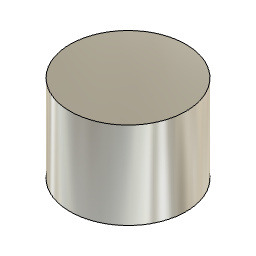
crane assembly v9 (Autodesk Fusion 360 archive; units mm, degrees)
design "electromagnet"
Autodesk Fusion 360 part; units mm, degrees
sketch "Sketch1" plane through (0, 0, 0) normal (0, 0, 1) x (1, 0, 0)
  circle A0 centre (0, 0) radius 10
  dimension "d1" = 20
  constraint coincident A0.centre origin
  measures "d1" diameter of A0
extrude "Extrude1" add sketch "Sketch1" along normal blind 15
sketch "Sketch2" plane through (0, 0, 0) normal (0, 0, -1) x (1, 0, 0)
  circle A0 centre (0, 0) radius 10
  circle A1 centre (0, 0) radius 2
  dimension "d4" = 4
  constraint concentric A0 A1
  measures "d4" diameter of A1
extrude "Extrude2" cut sketch "Sketch2" against normal blind 5 contours A1

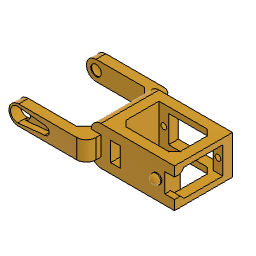
design "second link"
Autodesk Fusion 360 part; units mm, degrees
sketch "Sketch1" plane through (0, 0, 0) normal (0, 0, 1) x (1, 0, 0)
  line L0 (0, 0) -> (40, 0)
  line L1 (40, 0) -> (40, 5)
  line L2 (40, 5) -> (0, 5)
  line L3 (0, 5) -> (0, 0)
  dimension "d1" = 40
  dimension "d2" = 5
  constraint horizontal L0
  constraint vertical L1
  constraint horizontal L2
  constraint vertical L3
  constraint coincident L0.start L3.end
  measures "d1" distance of L0.start L0.end
  measures "d2" distance of L0.start L2.end
extrude "Extrude1" add sketch "Sketch1" along normal blind 10
sketch "Sketch3" plane through (0, 0, 0) normal (0, -1, 0) x (1, 0, 0)
  line L0 (0, 0) -> (40, 0)
  line L1 (40, 0) -> (40, 10)
  line L2 (40, 10) -> (0, 10)
  line L3 (0, 10) -> (0, 0)
  line L4 (0, 5) -> (4.5, 5) construction
  circle A0 centre (4.5, 5) radius 3.7
  line L5 (4.5, 5) -> (18.5, 5) construction
  circle A1 centre (18.5, 5) radius 2.25
  line L6 (18.5, 5) -> (18.5, 7.25) construction
  line L7 (18.5, 5) -> (18.5, 2.75) construction
  line L8 (4.5, 5) -> (4.5, 8.7) construction
  line L9 (4.5, 5) -> (4.5, 1.3) construction
  line L10 (4.5, 1.3) -> (18.5, 2.75)
  line L11 (4.5, 8.7) -> (18.5, 7.25)
  dimension "d5" = 4.5
  dimension "d6" = 7.4
  dimension "d7" = 14
  dimension "d8" = 4.5
  constraint midpoint L3 L4.start
  constraint perpendicular L3 L4
  constraint coincident L4.end A0.centre
  constraint parallel L4 L5
  constraint coincident L5.end A1.centre
  constraint coincident A1 L6.end
  constraint perpendicular L5 L6
  constraint coincident A1 L7.end
  constraint perpendicular L5 L7
  constraint coincident A0 L8.end
  constraint perpendicular L5 L8
  constraint coincident A0 L9.end
  constraint perpendicular L5 L9
  measures "d5" distance of L4.start L4.end
  measures "d6" diameter of A0
  measures "d7" distance of L4.end L5.end
  measures "d8" diameter of A1
extrude "Extrude2" cut sketch "Sketch3" against normal blind 5 contours A0 L10 L11
extrude "Extrude3" cut sketch "Sketch3" against normal blind 3 contours A0 A1 L10 L11 | A1
fillet "Fillet1" radius 5 2 edges at (0, 2.5, 10) (0, 2.5, 0)
sketch "Sketch4" plane through (0, 5, 0) normal (0, 1, 0) x (-1, 0, 0)
  arc A0 (-5.2583, 8.6215) -> (-5.2583, 1.3785) centre (-4.5, 5) ccw
  line L0 (-5.2583, 8.6215) -> (-4.5, 8.7)
  arc A1 (-4.5, 1.3) -> (-4.5, 8.7) centre (-4.5, 5) ccw
  line L1 (-4.5, 1.3) -> (-5.2583, 1.3785)
  arc A2 (-5, 0) -> (-5, 10) centre (-5, 5) ccw
  line L2 (-5, 10) -> (-40, 10)
  line L3 (-40, 10) -> (-40, 0)
  line L4 (-40, 0) -> (-5, 0)
  line L5 (-40, 0) -> (-35, 0)
  line L6 (-35, 0) -> (-35, 10)
  line L7 (-35, 10) -> (-40, 10)
  line L8 (-40, 10) -> (-40, 0)
  dimension "d15" = 5
  constraint horizontal L5
  constraint vertical L6
  constraint horizontal L7
  constraint vertical L8
  constraint coincident L3.end L4.start
  measures "d15" distance of L3.end L5.end
extrude "Extrude4" add sketch "Sketch4" along normal blind 40 contours L2 L3 L4 L5 L6 L7 L8
sketch "Sketch5" plane through (35, 0, 0) normal (-1, 0, 0) x (0, -1, 0)
  line L0 (-5, 0) -> (-5, 10)
  line L1 (-5, 10) -> (-45, 10)
  line L2 (-45, 10) -> (-45, 0)
  line L3 (-45, 0) -> (-5, 0)
  line L4 (-45, 10) -> (-40, 10)
  line L5 (-40, 10) -> (-40, 0)
  line L6 (-40, 0) -> (-45, 0)
  line L7 (-45, 0) -> (-45, 10)
  dimension "d18" = 5
  constraint horizontal L4
  constraint vertical L5
  constraint horizontal L6
  constraint vertical L7
  constraint coincident L1.end L2.start
  measures "d18" distance of L1.end L4.end
extrude "Extrude5" add sketch "Sketch5" along normal blind 35 contours L1 L2 L3 L4 L5 L6 L7
sketch "Sketch6" plane through (0, 40, 0) normal (0, -1, 0) x (1, 0, 0)
  line L0 (35, 0) -> (35, 10)
  line L1 (35, 10) -> (0, 10)
  line L2 (0, 10) -> (0, 0)
  line L3 (0, 0) -> (35, 0)
  line L4 (0, 5) -> (5, 5) construction
  circle A0 centre (5, 5) radius 2.75
  dimension "d21" = 5
  dimension "d22" = 5.5
  constraint midpoint L2 L4.start
  constraint perpendicular L2 L4
  constraint coincident L4.end A0.centre
  measures "d21" distance of L4.start L4.end
  measures "d22" diameter of A0
extrude "Extrude6" cut sketch "Sketch6" against normal blind 3 contours A0
fillet "Fillet2" radius 2.5 1 edges at (2.4361, 43, 5.9944)
fillet "Fillet3" radius 5 2 edges at (0, 42.5, 10) (0, 42.5, 0)
chamfer "Chamfer1" distance 5 angle 45 2 edges at (35, 40, 5) (35, 5, 5)
sketch "Sketch7" plane through (40, 0, 0) normal (1, 0, 0) x (0, 1, 0)
  line L0 (0, 0) -> (45, 0)
  line L1 (45, 0) -> (45, 10)
  line L2 (45, 10) -> (0, 10)
  line L3 (0, 10) -> (0, 0)
  line L4 (45, 10) -> (32.5, 10) construction
  line L5 (32.5, 10) -> (12.5, 10)
  line L6 (12.5, 10) -> (12.5, 0)
  line L7 (12.5, 0) -> (32.5, 0)
  line L8 (32.5, 0) -> (32.5, 10)
  line L9 (32.5, 10) -> (12.5, 10)
  line L10 (12.5, 10) -> (12.5, 15)
  line L11 (12.5, 15) -> (32.5, 15)
  line L12 (32.5, 15) -> (32.5, 10)
  line L13 (32.5, 0) -> (12.5, 0)
  line L14 (12.5, 0) -> (12.5, -5)
  line L15 (12.5, -5) -> (32.5, -5)
  line L16 (32.5, -5) -> (32.5, 0)
  line L17 (32.5, -5) -> (37.5, -5)
  line L18 (37.5, -5) -> (37.5, 15)
  line L19 (37.5, 15) -> (32.5, 15)
  line L20 (32.5, 15) -> (32.5, -5)
  line L21 (12.5, -5) -> (7.5, -5)
  line L22 (7.5, -5) -> (7.5, 15)
  line L23 (7.5, 15) -> (12.5, 15)
  line L24 (12.5, 15) -> (12.5, -5)
  dimension "d30" = 12.5
  dimension "d31" = 20
  dimension "d32" = 5
  dimension "d33" = 20
  dimension "d34" = 5
  dimension "d35" = 5
  dimension "d36" = 20
  dimension "d37" = 5
  dimension "d38" = 20
  constraint coincident L1.end L2.start
  constraint perpendicular L1 L4
  constraint horizontal L5
  constraint vertical L6
  constraint horizontal L7
  constraint vertical L8
  constraint coincident L0 L6.end
  constraint horizontal L9
  constraint vertical L10
  constraint horizontal L11
  constraint vertical L12
  constraint horizontal L13
  constraint vertical L14
  constraint horizontal L15
  constraint vertical L16
  constraint horizontal L17
  constraint vertical L18
  constraint horizontal L19
  constraint vertical L20
  constraint horizontal L21
  constraint vertical L22
  constraint horizontal L23
  constraint vertical L24
  measures "d30" distance of L1.end L4.end
  measures "d31" distance of L4.end L5.end
  measures "d32" distance of L4.end L11.end
  measures "d33" distance of L7.end L6.end
  measures "d34" distance of L7.end L15.end
  measures "d35" distance of L15.end L17.end
  measures "d36" distance of L15.end L11.end
  measures "d37" distance of L14.end L21.end
  measures "d38" distance of L14.end L10.end
extrude "Extrude7" add sketch "Sketch7" along normal blind 5 contours L0 L2 L5 L6 L7 L8 L9 L13 L20 L24 | L0 L14 L21 L22 L24 | L0 L2 L6 L22 L24 | L0 L7 L13 L14 L15 L16 L20 L24 | L0 L2 L8 L18 L20 | L0 L16 L17 L18 L20 | L2 L5 L9 L10 L11 L12 L20 L24 | L2 L10 L22 L23 L24 | L2 L12 L18 L19 L20
revolve "Revolve1" add 2 faces at (40, 17.5, 13.3333) (40, 17.5, 13.3333) angle 360 about axis through (40, 0, 10) along (0, 1, 0)
revolve "Revolve2" add 2 faces at (40, 17.5, -1.6667) (40, 17.5, -1.6667) angle 360 about axis through (40, 0, 0) along (0, 1, 0)
sketch "Sketch8" plane through (45, 0, 0) normal (1, 0, 0) x (0, 1, 0)
  line L0 (37.5, -5) -> (37.5, 15)
  line L1 (37.5, 15) -> (7.5, 15)
  line L2 (7.5, 15) -> (7.5, -5)
  line L3 (7.5, -5) -> (37.5, -5)
  line L4 (37.5, 15) -> (32.5, 15)
  line L5 (32.5, 15) -> (32.5, 12)
  line L6 (32.5, 12) -> (37.5, 12)
  line L7 (37.5, 12) -> (37.5, 15)
  line L8 (37.5, -5) -> (32.5, -5)
  line L9 (32.5, -5) -> (32.5, -2)
  line L10 (32.5, -2) -> (37.5, -2)
  line L11 (37.5, -2) -> (37.5, -5)
  line L12 (7.5, -5) -> (12.5, -5)
  line L13 (12.5, -5) -> (12.5, 0)
  line L14 (12.5, 0) -> (7.5, 0)
  line L15 (7.5, 0) -> (7.5, -5)
  line L16 (7.5, 15) -> (12.5, 15)
  line L17 (12.5, 15) -> (12.5, 10)
  line L18 (12.5, 10) -> (7.5, 10)
  line L19 (7.5, 10) -> (7.5, 15)
  dimension "d43" = 5
  dimension "d44" = 3
  dimension "d45" = 5
  dimension "d46" = 3
  dimension "d47" = 5
  dimension "d48" = 5
  dimension "d49" = 5
  dimension "d50" = 5
  constraint horizontal L4
  constraint vertical L5
  constraint horizontal L6
  constraint vertical L7
  constraint coincident L0.end L1.start
  constraint horizontal L8
  constraint vertical L9
  constraint horizontal L10
  constraint vertical L11
  constraint coincident L0.start L3.end
  constraint horizontal L12
  constraint vertical L13
  constraint horizontal L14
  constraint vertical L15
  constraint coincident L2.end L3.start
  constraint horizontal L16
  constraint vertical L17
  constraint horizontal L18
  constraint vertical L19
  constraint coincident L1.end L2.start
  measures "d43" distance of L0.end L4.end
  measures "d44" distance of L0.end L6.end
  measures "d45" distance of L0.start L8.end
  measures "d46" distance of L0.start L10.end
  measures "d47" distance of L2.end L12.end
  measures "d48" distance of L2.end L14.end
  measures "d49" distance of L1.end L16.end
  measures "d50" distance of L1.end L18.end
extrude "Extrude8" add sketch "Sketch8" along normal blind 33 contours L0 L3 L8 L9 L10 L11 | L0 L1 L4 L5 L6 L7 | L2 L3 L12 L13 L14 L15 | L1 L2 L16 L17 L18 L19
sketch "Sketch9" plane through (0, 0, -2) normal (0, 0, 1) x (-1, 0, 0)
  line L0 (-45, -37.5) -> (-45, -32.5)
  line L1 (-45, -32.5) -> (-78, -32.5)
  line L2 (-78, -32.5) -> (-78, -37.5)
  line L3 (-78, -37.5) -> (-45, -37.5)
  line L4 (-45, -32.5) -> (-50, -32.5)
  line L5 (-50, -32.5) -> (-50, -37.5)
  line L6 (-50, -37.5) -> (-45, -37.5)
  line L7 (-45, -37.5) -> (-45, -32.5)
  line L8 (-78, -37.5) -> (-73, -37.5)
  line L9 (-73, -37.5) -> (-73, -32.5)
  line L10 (-73, -32.5) -> (-78, -32.5)
  line L11 (-78, -32.5) -> (-78, -37.5)
  dimension "d53" = 5
  dimension "d54" = 5
  dimension "d55" = 5
  dimension "d56" = 5
  constraint horizontal L4
  constraint vertical L5
  constraint horizontal L6
  constraint vertical L7
  constraint coincident L0.end L1.start
  constraint horizontal L8
  constraint vertical L9
  constraint horizontal L10
  constraint vertical L11
  constraint coincident L2.end L3.start
  measures "d53" distance of L0.end L4.end
  measures "d54" distance of L0.end L0.start
  measures "d55" distance of L2.end L8.end
  measures "d56" distance of L2.end L1.end
extrude "Extrude9" add sketch "Sketch9" along normal blind 14 contours L0 L1 L3 L4 L5 L6 L7 | L1 L2 L3 L8 L9 L10 L11
sketch "Sketch10" plane through (0, 32.5, 0) normal (0, -1, 0) x (1, 0, 0)
  line L0 (73, 12) -> (73, -2)
  line L1 (73, -2) -> (50, -2)
  line L2 (50, -2) -> (50, 12)
  line L3 (45, 15) -> (45, -5)
  line L4 (45, -5) -> (78, -5)
  line L5 (78, -5) -> (78, 15)
  line L6 (45, 5) -> (47.5, 5)
  circle A0 centre (47.5, 5) radius 1.5
  line L7 (73, 5) -> (75.5, 5)
  circle A1 centre (75.5, 5) radius 1.5
  line L8 (50, 12) -> (73, 12)
  line L9 (78, 15) -> (45, 15)
  dimension "d59" = 2.5
  dimension "d60" = 3
  dimension "d61" = 2.5
  dimension "d62" = 3
  constraint midpoint L3 L6.start
  constraint perpendicular L2 L6
  constraint coincident L6.end A0.centre
  constraint midpoint L0 L7.start
  constraint perpendicular L5 L7
  constraint coincident L7.end A1.centre
  measures "d59" distance of L6.start L6.end
  measures "d60" diameter of A0
  measures "d61" distance of L7.start L7.end
  measures "d62" diameter of A1
extrude "Extrude10" cut sketch "Sketch10" against normal blind 5 contours A0 | A1
sketch "Sketch11" plane through (0, 32.5, 0) normal (0, -1, 0) x (1, 0, 0)
  circle A0 centre (47.5, 5) radius 1.5
  circle A1 centre (75.5, 5) radius 1.5
  line L0 (73, 12) -> (73, -2)
  line L1 (73, -2) -> (50, -2)
  line L2 (50, -2) -> (50, 12)
  line L3 (45, 15) -> (45, -5)
  line L4 (45, -5) -> (78, -5)
  line L5 (78, -5) -> (78, 15)
  line L6 (78, 15) -> (73, 15)
  line L7 (73, 15) -> (73, 12)
  line L8 (73, 12) -> (78, 12)
  line L9 (78, 12) -> (78, 15)
  line L10 (78, -5) -> (73, -5)
  line L11 (73, -5) -> (73, -2)
  line L12 (73, -2) -> (78, -2)
  line L13 (78, -2) -> (78, -5)
  line L14 (50, 12) -> (73, 12)
  line L15 (78, 15) -> (45, 15)
  dimension "d69" = 5
  dimension "d70" = 3
  dimension "d71" = 5
  dimension "d72" = 3
  constraint horizontal L6
  constraint vertical L7
  constraint horizontal L8
  constraint vertical L9
  constraint coincident L5.end L6.start
  constraint horizontal L10
  constraint vertical L11
  constraint horizontal L12
  constraint vertical L13
  constraint coincident L4.end L5.start
  measures "d69" distance of L5.end L6.end
  measures "d70" distance of L5.end L8.end
  measures "d71" distance of L4.end L10.end
  measures "d72" distance of L4.end L12.end
extrude "Extrude11" add sketch "Sketch11" along normal blind 20 contours L5 L6 L7 L8 L9 L15 | L4 L5 L10 L11 L12 L13
sketch "Sketch12" plane through (0, 0, 0) normal (0, 0, 1) x (-1, 0, 0)
  line L0 (-45, -12.5) -> (-45, -7.5)
  line L1 (-45, -7.5) -> (-78, -7.5)
  line L2 (-78, -7.5) -> (-78, -12.5)
  line L3 (-78, -12.5) -> (-45, -12.5)
  line L4 (-78, -7.5) -> (-73, -7.5) construction
  line L5 (-73, -7.5) -> (-73, -12.5) construction
  line L6 (-73, -12.5) -> (-78, -12.5) construction
  line L7 (-78, -12.5) -> (-78, -7.5) construction
  line L8 (-45, -7.5) -> (-50, -7.5) construction
  line L9 (-50, -7.5) -> (-50, -12.5) construction
  line L10 (-50, -12.5) -> (-45, -12.5) construction
  line L11 (-45, -12.5) -> (-45, -7.5) construction
  line L12 (-73, -7.5) -> (-50, -7.5)
  line L13 (-50, -7.5) -> (-50, -12.5)
  line L14 (-50, -12.5) -> (-73, -12.5)
  line L15 (-73, -12.5) -> (-73, -7.5)
  dimension "d75" = 5
  dimension "d76" = 5
  constraint horizontal L4
  constraint vertical L5
  constraint horizontal L6
  constraint vertical L7
  constraint coincident L1.end L2.start
  constraint horizontal L8
  constraint vertical L9
  constraint horizontal L10
  constraint vertical L11
  constraint coincident L0.end L1.start
  constraint horizontal L12
  constraint vertical L13
  constraint horizontal L14
  constraint vertical L15
  measures "d75" distance of L1.end L4.end
  measures "d76" distance of L0.end L8.end
extrude "Extrude12" add sketch "Sketch12" along normal blind 10 contours L1 L3 L12 L13 L14 L15
chamfer "Chamfer2" distance 2 angle 45 2 edges at (75.5, 12.5, 0) (75.5, 12.5, 10)
chamfer "Chamfer3" distance 3 angle 45 6 edges at (73, 12.5, 13.5) (73, 32.5, 13.5) (45, 12.5, 12.5) (45, 12.5, -2.5) (73, 32.5, -3.5) (73, 12.5, -3.5)
fillet "Fillet4" radius 5 2 edges at (40, 0, 5) (40, 45, 5)
sketch "Sketch13" plane through (0, 7.5, 0) normal (0, -1, 0) x (1, 0, 0)
  line L0 (73, 10) -> (78, 10)
  line L1 (78, 10) -> (78, 15)
  line L2 (78, 15) -> (40, 15)
  arc A0 (40, 15) -> (35, 10) centre (40, 10) ccw
  line L3 (35, 10) -> (40, 10)
  line L4 (40, 10) -> (40, 0)
  line L5 (40, 0) -> (35, 0)
  arc A1 (35, 0) -> (40, -5) centre (40, 0) ccw
  line L6 (40, -5) -> (78, -5)
  line L7 (78, -5) -> (78, 0)
  line L8 (78, 0) -> (73, 0)
  line L9 (73, 0) -> (73, 10)
  line L10 (50, 10) -> (50, 0)
  line L11 (50, 0) -> (45, 0)
  line L12 (45, 0) -> (45, 10)
  line L13 (45, 10) -> (50, 10)
  line L14 (73, 5) -> (69, 5) construction
  circle A2 centre (69, 5) radius 2.5
  dimension "d83" = 4
  dimension "d84" = 5
  constraint midpoint L9 L14.start
  constraint perpendicular L9 L14
  constraint coincident L14.end A2.centre
  measures "d83" distance of L14.start L14.end
  measures "d84" diameter of A2
extrude "Extrude13" add sketch "Sketch13" along normal blind 3 contours A2
fillet "Fillet5" radius 2.5 1 edges at (66.6692, 4.5, 4.096)

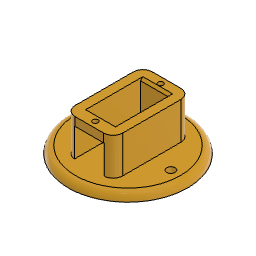
design "crane_base"
Autodesk Fusion 360 part; units mm, degrees
sketch "Sketch1" plane through (0, 0, 0) normal (0, 0, 1) x (1, 0, 0)
  circle A0 centre (0, 0) radius 25
  line L0 (0, 0) -> (-18, 0) construction
  line L1 (0, 0) -> (18, 0) construction
  circle A1 centre (-18, 0) radius 1.75
  circle A2 centre (18, 0) radius 1.75
  dimension "d1" = 50
  dimension "d25" = 18
  dimension "d26" = 18
  dimension "d27" = 3.5
  dimension "d28" = 3.5
  constraint coincident A0.centre L0.start
  constraint horizontal L0
  constraint parallel L0 L1
  constraint coincident L0.end A1.centre
  constraint coincident L1.end A2.centre
  measures "d1" diameter of A0
  measures "d25" distance of A0.centre L0.end
  measures "d26" distance of A0.centre L1.end
  measures "d27" diameter of A1
  measures "d28" diameter of A2
extrude "Extrude1" add sketch "Sketch1" along normal blind 3
sketch "Sketch2" plane through (0, 0, 3) normal (0, 0, 1) x (-1, 0, 0)
  circle A0 centre (0, 0) radius 25
  line L0 (-6.25, 11.5) -> (6.25, 11.5)
  line L1 (6.25, 11.5) -> (6.25, -11.5)
  line L2 (6.25, -11.5) -> (-6.25, -11.5)
  line L3 (-6.25, -11.5) -> (-6.25, 11.5)
  line L4 (-6.25, 11.5) -> (6.25, -11.5) construction
  line L5 (6.25, 11.5) -> (-6.25, -11.5) construction
  line L6 (-10, -16.225) -> (10, -16.225)
  line L7 (10, -16.225) -> (10, 16.225)
  line L8 (10, 16.225) -> (-10, 16.225)
  line L9 (-10, 16.225) -> (-10, -16.225)
  line L10 (-10, -16.225) -> (10, 16.225) construction
  line L11 (10, -16.225) -> (-10, 16.225) construction
  circle A1 centre (-18, 0) radius 1.75
  circle A2 centre (18, 0) radius 1.75
  dimension "d4" = 12.5
  dimension "d5" = 23
  dimension "d6" = 20
  dimension "d7" = 32.45
  constraint horizontal L0
  constraint perpendicular L0 L1
  constraint parallel L0 L2
  constraint parallel L1 L3
  constraint coincident L4 A0.centre
  constraint coincident L5 A0.centre
  constraint coincident A0.centre origin
  constraint horizontal L6
  constraint perpendicular L6 L7
  constraint parallel L6 L8
  constraint parallel L7 L9
  constraint coincident L10 A0.centre
  constraint coincident L11 A0.centre
  measures "d4" distance of L1.end L2.end
  measures "d5" distance of L0.end L1.end
  measures "d6" distance of L7.end L8.end
  measures "d7" distance of L6.end L7.end
extrude "Extrude2" add sketch "Sketch2" along normal blind 15.55 contours L6 L7 L8 L9
sketch "Sketch3" plane through (0, 0, 18.55) normal (0, 0, 1) x (-1, 0, 0)
  line L0 (6.25, -11.5) -> (-6.25, -11.5)
  line L1 (-6.25, -11.5) -> (-6.25, 11.5)
  line L2 (-6.25, 11.5) -> (6.25, 11.5)
  line L3 (6.25, 11.5) -> (6.25, -11.5)
  line L4 (-10, 16.225) -> (-10, -16.225)
  line L5 (-10, -16.225) -> (10, -16.225)
  line L6 (10, -16.225) -> (10, 16.225)
  line L7 (10, 16.225) -> (-10, 16.225)
  line L8 (0, 16.225) -> (0, 13.667) construction
  line L9 (0, -16.225) -> (0, -13.667) construction
  circle A0 centre (0, -13.667) radius 1.1
  circle A1 centre (0, 13.667) radius 1.1
  dimension "d10" = 2.558
  dimension "d11" = 2.558
  dimension "d12" = 2.2
  dimension "d13" = 2.2
  constraint midpoint L7 L8.start
  constraint perpendicular L7 L8
  constraint midpoint L5 L9.start
  constraint perpendicular L5 L9
  constraint coincident L9.end A0.centre
  constraint coincident L8.end A1.centre
  measures "d10" distance of L8.start L8.end
  measures "d11" distance of L9.start L9.end
  measures "d12" diameter of A0
  measures "d13" diameter of A1
extrude "Extrude3" cut sketch "Sketch3" against normal blind 10 contours A0 | A1
sketch "Sketch4" plane through (0, -16.225, 0) normal (0, -1, 0) x (1, 0, 0)
  line L0 (-10, 3) -> (10, 3)
  line L1 (10, 3) -> (10, 18.55)
  line L2 (10, 18.55) -> (-10, 18.55)
  line L3 (-10, 18.55) -> (-10, 3)
  line L4 (0, 3) -> (-6.25, 3) construction
  line L5 (-6.25, 3) -> (6.25, 3)
  line L6 (6.25, 3) -> (6.25, 15)
  line L7 (6.25, 15) -> (-6.25, 15)
  line L8 (-6.25, 15) -> (-6.25, 3)
  dimension "d16" = 6.25
  dimension "d17" = 12.5
  dimension "d18" = 12
  constraint midpoint L0 L4.start
  constraint parallel L0 L4
  constraint horizontal L5
  constraint vertical L6
  constraint horizontal L7
  constraint vertical L8
  measures "d16" distance of L4.start L4.end
  measures "d17" distance of L4.end L5.end
  measures "d18" distance of L4.end L7.end
extrude "Extrude4" cut sketch "Sketch4" against normal blind 4.725 contours L0 L5 L6 L7 L8
fillet "Fillet2" radius 4 4 edges at (10, -16.225, 10.775) (10, 16.225, 10.775) (-10, 16.225, 10.775) (-10, -16.225, 10.775)
fillet "Fillet3" radius 3 1 edges at (-23.3082, -9.0404, 3)
chamfer "Chamfer1" distance 2 angle 45 1 edges at (0, -11.5, 15)
chamfer "Chamfer2" distance 1 angle 45 1 edges at (0, 11.5, 18.55)

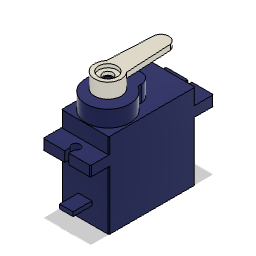
design "SG90 9g servo"
Autodesk Fusion 360 part; units mm, degrees
sketch "Body" plane through (0, 0, 0) normal (0, 1, 0) x (1, 0, 0) in component "servo"
  line L0 (6.25, -11.375) -> (-6.25, -11.375)
  line L1 (-6.25, -11.375) -> (-6.25, 11.375)
  line L2 (-6.25, 11.375) -> (6.25, 11.375)
  line L3 (6.25, 11.375) -> (6.25, -11.375)
  line L4 (6.25, -11.375) -> (-6.25, 11.375) construction
  line L5 (-6.25, -11.375) -> (6.25, 11.375) construction
  dimension "d6" = 12.5
  dimension "d7" = 22.75
  dimension "d52" = 0
  dimension "d53" = 0
  dimension "d54" = 0
  dimension "d55" = 0
  constraint perpendicular L0 L1
  constraint parallel L0 L2
  constraint parallel L1 L3
  constraint horizontal L0
  constraint coincident L4 origin
  constraint coincident L5 origin
  measures "d6" distance of L1.end L2.end
  measures "d7" distance of L0.end L1.end
extrude "Extrude1" add sketch "Body" along normal blind 22.35 makes body 1 in component "servo"
sketch "Tab" plane through (0, 0, 11.375) normal (0, 0, 1) x (1, 0, 0) in component "servo"
  line L0 (-6.25, 0) -> (6.25, 0)
  line L1 (6.25, 0) -> (6.25, 22.35)
  line L2 (6.25, 22.35) -> (-6.25, 22.35)
  line L3 (-6.25, 22.35) -> (-6.25, 0)
  line L4 (-6.25, 18.2) -> (6.25, 18.2)
  line L5 (6.25, 18.2) -> (6.25, 15.55)
  line L6 (6.25, 15.55) -> (-6.25, 15.55)
  line L7 (-6.25, 15.55) -> (-6.25, 18.2)
  dimension "d10" = 4.15
  dimension "d11" = 2.65
  constraint horizontal L4
  constraint vertical L5
  constraint horizontal L6
  constraint vertical L7
  constraint coincident L1 L5.end
  constraint coincident L3 L4.start
  measures "d10" distance of L1.end L4.end
  measures "d11" distance of L4.end L5.end
extrude "Extrude2" add sketch "Tab" along normal blind 4.85 contours L1 L3 L4 L5 L6 L7 bodies 1 in component "servo"
hole "Hole1" at (0, 18.2, 13.8) direction (0, -1, 0) diameter 2.2 end through all bodies 1 in component "servo"
fillet "Fillet1" radius 0.25 2 edges at (6.25, 16.875, 16.225) (-6.25, 16.875, 16.225) on bodies 1 in component "servo"
sketch "Notch" plane through (0, 0, 16.225) normal (0, 0, 1) x (1, 0, 0) in component "servo"
  line L0 (-6, 18.2) -> (-6, 15.55)
  line L1 (-6, 15.55) -> (6, 15.55)
  line L2 (6, 15.55) -> (6, 18.2)
  line L3 (6, 18.2) -> (-6, 18.2)
  line L4 (-0.525, 18.2) -> (0.525, 18.2)
  line L5 (0.525, 18.2) -> (0.525, 15.55)
  line L6 (0.525, 15.55) -> (-0.525, 15.55)
  line L7 (-0.525, 15.55) -> (-0.525, 18.2)
  dimension "d20" = 1.05
  constraint collinear L3 L4
  constraint collinear L1 L6
  constraint parallel L5 L7
  measures "d20" distance of L4.start L4.end
extrude "Extrude3" cut sketch "Notch" along normal up to surface contours L1 L3 L4 L5 L6 L7 end surface at (0.0548, 17.3167, 14.8986) on bodies 1 bodies 1 in component "servo"
mirror "Mirror1" about plane through (0, 0, 0) normal (0, 0, 1) of "Extrude2", "Hole1", "Fillet1", "Extrude3" in component "servo"
sketch "Bump" plane through (0, 22.35, 0) normal (0, 1, 0) x (-1, 0, 0) in component "servo"
  line L0 (-6.25, -11.375) -> (6.25, -11.375)
  line L1 (6.25, -11.375) -> (6.25, 11.375)
  line L2 (6.25, 11.375) -> (-6.25, 11.375)
  line L3 (-6.25, 11.375) -> (-6.25, -11.375)
  line L4 (-2.8, -0.625) -> (-2.8, 0.2671)
  line L5 (2.8, 0.2671) -> (2.8, -0.625)
  arc A0 (-2.8, -0.625) -> (2.8, -0.625) centre (0, -0.625) ccw
  arc A1 (2.8, 0.2671) -> (-2.8, 0.2671) centre (0, 5.375) ccw
  dimension "d23" = 11.65
  dimension "d24" = 6
  dimension "d25" = 5.6
  dimension "d26" = 6
  dimension "d27" = 6.25
  dimension "d28" = 6.25
  constraint tangent L4 A0
  constraint vertical L4
  constraint tangent L5 A0
  measures "d23" diameter of A1
  measures "d24" distance of L2 A1.centre
  measures "d25" diameter of A0
  measures "d26" distance of A1.centre A0.centre
  measures "d27" distance of L3 A1.centre
  measures "d28" distance of L3 A0.centre
extrude "Extrude4" add sketch "Bump" along normal blind 4.3 contours L4 L5 A0 A1 bodies 1 in component "servo"
fillet "Fillet2" radius 0.25 8 edges at (6.25, 7.775, 11.375) (6.25, 20.275, 11.375) (-6.25, 20.275, 11.375) (-6.25, 7.775, 11.375) (6.25, 7.775, -11.375) (6.25, 20.275, -11.375) (-6.25, 20.275, -11.375) (-6.25, 7.775, -11.375) on bodies 1 in component "servo"
hole "Hole2" at (0, 26.65, 5.375) direction (0, -1, 0) diameter 4.92 depth 15 tip angle 180 bodies 1 in component "servo"
sketch "Wire" plane through (0, 0, 11.375) normal (0, 0, 1) x (1, 0, 0) in component "servo"
  line L0 (-6, 15.55) -> (-6, 0)
  line L1 (-6, 0) -> (6, 0)
  line L2 (6, 0) -> (6, 15.55)
  line L3 (6, 15.55) -> (-6, 15.55)
  line L4 (-1.8, 5.5) -> (1.8, 5.5)
  line L5 (1.8, 5.5) -> (1.8, 4.4)
  line L6 (1.8, 4.4) -> (-1.8, 4.4)
  line L7 (-1.8, 4.4) -> (-1.8, 5.5)
  dimension "d32" = 1.1
  dimension "d33" = 3.6
  dimension "d34" = 5.5
  constraint horizontal L4
  constraint vertical L5
  constraint horizontal L6
  constraint vertical L7
  measures "d32" distance of L4.start L6.end
  measures "d33" distance of L4.start L4.end
  measures "d34" distance of L1 L4.end
extrude "Extrude5" add sketch "Wire" along normal blind 5 contours L4 L5 L6 L7 bodies 1 in component "servo"
cylinder "CylinderPrimitive1" add diameter 4.92 height 2.72 placed x (1, 0, 0) y (0, 0, -1) z (0, 1, 0) at (0, 26.65, 5.375) separate body makes body 2 in component "splined-drive"
extrude "Extrude1'" add 1 faces at (-0.4548, 26.65, 5.9711) along direction (0, -1, 0) blind 15 on bodies 2 bodies 2 in component "splined-drive"
hole "Hole1'" at (0, 29.37, 5.375) direction (0, -1, 0) diameter 1.95 depth 5 tip angle 180 bodies 2 in component "splined-drive"
chamfer "Chamfer1" distance 0.25 angle 45 1 edges at (-2.2935, 29.37, 6.2646) on bodies 2 in component "splined-drive"
sketch "Sketch1" plane through (0, 29.37, 0) normal (0, 1, 0) x (-1, 0, 0) in component "horn"
  circle A0 centre (0, 5.375) radius 3.5
  circle A1 centre (0, 5.375) radius 2.46
  circle A2 centre (0, 5.375) radius 1.31
  dimension "d102" = 0
  dimension "d103" = 0
  dimension "d104" = 0
  dimension "d105" = 0
extrude "Extrude3'" add sketch "Sketch1" against normal blind 2.08 separate body contours A0 makes body 3 in component "horn"
extrude "Extrude6" add 1 faces at (-3.1311, 29.37, 5.0789) along direction (0, 1, 0) blind 1.83 on bodies 3 bodies 3 in component "horn"
extrude "Extrude4'" add sketch "Sketch1" along normal blind 0.9 contours A1 bodies 3 in component "horn"
sketch "Sketch4" plane through (0, 31.2, 0) normal (0, 1, 0) x (-1, 0, 0) in component "horn"
  circle A0 centre (0, 5.375) radius 2.46
  circle A1 centre (0, 5.375) radius 3.5
  line L0 (2.67, 3.112) -> (2.04, -9.105)
  line L1 (-2.67, 3.112) -> (-2.04, -9.105)
  arc A2 (-2.04, -9.105) -> (2.04, -9.105) centre (0, -8.6045) ccw
  constraint coincident A1 L0.start
  constraint coincident A1 L1.start
extrude "Extrude7" add sketch "Sketch4" against normal blind 1.41 contours A1 L0 L1 A2 bodies 3 in component "horn"
component "servo" placed x (1, 0, 0) y (0, 1, 0) z (0, 0, 1) at (0, 0, 0)
component "splined-drive" placed x (1, 0, 0) y (0, 1, 0) z (0, 0, 1) at (0, 0, 0)
component "horn" placed x (1, 0, 0) y (0, 1, 0) z (0, 0, 1) at (0, 0, 0)

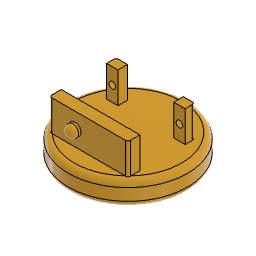
design "first crane stand"
part number: Configuration 1
Autodesk Fusion 360 part; units mm, degrees
sketch "Sketch1" plane through (0, 0, 0) normal (0, 0, 1) x (1, 0, 0)
  circle A0 centre (0, 0) radius 25
  dimension "d1" = 50
  constraint coincident A0.centre origin
  measures "d1" diameter of A0
extrude "Extrude1" add sketch "Sketch1" along normal blind 10
sketch "Sketch2" plane through (0, 0, 0) normal (0, 0, -1) x (1, 0, 0)
  circle A0 centre (0, 0) radius 25
  line L0 (0, 0) -> (0, -10) construction
  circle A1 centre (0, -10) radius 3.5
  line L1 (0, -10) -> (0, -7.737) construction
  line L2 (0, -7.737) -> (-2.67, -7.737) construction
  line L3 (0, -7.737) -> (2.67, -7.737) construction
  line L4 (0, -10) -> (0, 3.98) construction
  circle A2 centre (0, 3.98) radius 2.1005
  line L5 (2.67, -7.737) -> (2.098, 4.0815)
  line L6 (-2.67, -7.737) -> (-2.098, 4.0815)
  dimension "d4" = 10
  dimension "d5" = 7
  dimension "d6" = 2.263
  dimension "d7" = 13.98
  dimension "d8" = 4.201
  constraint coincident A0.centre L0.start
  constraint vertical L0
  constraint coincident L0.end A1.centre
  constraint parallel L0 L1
  constraint coincident A1 L2.end
  constraint perpendicular L0 L2
  constraint coincident A1 L3.end
  constraint perpendicular L1 L3
  constraint parallel L0 L4
  constraint coincident L4.end A2.centre
  constraint coincident A2 L5.end
  constraint tangent A2 L5
  constraint coincident A2 L6.end
  constraint tangent A2 L6
  measures "d4" distance of A0.centre L0.end
  measures "d5" diameter of A1
  measures "d6" distance of L0.end L1.end
  measures "d7" distance of L0.end L4.end
  measures "d8" diameter of A2
extrude "Extrude2" cut sketch "Sketch2" against normal blind 2 contours A1 | A1 A2 L5 L6 | A2
sketch "Sketch14" plane through (0, 0, 10) normal (0, 0, 1) x (-1, 0, 0)
  circle A0 centre (0, 0) radius 25
  line L0 (16.5, 11.5) -> (-16.5, 11.5) construction
  line L1 (-16.5, 11.5) -> (-16.5, -11.5) construction
  line L2 (-16.5, -11.5) -> (16.5, -11.5) construction
  line L3 (16.5, -11.5) -> (16.5, 11.5) construction
  line L4 (16.5, 11.5) -> (-16.5, -11.5) construction
  line L5 (-16.5, 11.5) -> (16.5, -11.5) construction
  line L6 (-16.5, -11.5) -> (-11.7, -11.5)
  line L7 (-11.7, -11.5) -> (-11.7, -7.5)
  line L8 (-11.7, -7.5) -> (-16.5, -7.5)
  line L9 (-16.5, -7.5) -> (-16.5, -11.5)
  line L10 (16.5, -11.5) -> (11.7, -11.5)
  line L11 (11.7, -11.5) -> (11.7, -7.5)
  line L12 (11.7, -7.5) -> (16.5, -7.5)
  line L13 (16.5, -7.5) -> (16.5, -11.5)
  line L14 (16.5, 11.5) -> (-16.5, 11.5)
  line L15 (-16.5, 11.5) -> (-16.5, 16.5)
  line L16 (-16.5, 16.5) -> (16.5, 16.5)
  line L17 (16.5, 16.5) -> (16.5, 11.5)
  dimension "d95" = 33
  dimension "d96" = 23
  dimension "d97" = 4.8
  dimension "d98" = 4
  dimension "d99" = 4.8
  dimension "d100" = 4
  dimension "d101" = 33
  dimension "d102" = 5
  constraint horizontal L0
  constraint perpendicular L0 L1
  constraint parallel L0 L2
  constraint parallel L1 L3
  constraint coincident L4 A0.centre
  constraint coincident L5 A0.centre
  constraint coincident A0.centre origin
  constraint horizontal L6
  constraint vertical L7
  constraint horizontal L8
  constraint vertical L9
  constraint horizontal L10
  constraint vertical L11
  constraint horizontal L12
  constraint vertical L13
  constraint horizontal L14
  constraint vertical L15
  constraint horizontal L16
  constraint vertical L17
  measures "d95" distance of L1.end L2.end
  measures "d96" distance of L0.end L1.end
  measures "d97" distance of L1.end L6.end
  measures "d98" distance of L1.end L8.end
  measures "d99" distance of L2.end L10.end
  measures "d100" distance of L2.end L12.end
  measures "d101" distance of L0.start L0.end
  measures "d102" distance of L0.start L16.end
extrude "Extrude15" add sketch "Sketch14" along normal blind 13 contours L6 L7 L8 L9 | L10 L11 L12 L13 | L14 L15 L16 L17
sketch "Sketch15" plane through (0, 11.5, 0) normal (0, 1, 0) x (-1, 0, 0)
  line L0 (-16.5, 10) -> (-11.7, 10)
  line L1 (-11.7, 10) -> (-11.7, 23)
  line L2 (-11.7, 23) -> (-16.5, 23)
  line L3 (-16.5, 23) -> (-16.5, 10)
  line L4 (-14.1, 10) -> (-14.1, 16.25) construction
  circle A0 centre (-14.1, 16.25) radius 1.4
  dimension "d105" = 6.25
  dimension "d106" = 2.8
  constraint midpoint L0 L4.start
  constraint perpendicular L0 L4
  constraint coincident L4.end A0.centre
  measures "d105" distance of L4.start L4.end
  measures "d106" diameter of A0
sketch "Sketch16" plane through (0, 11.5, 0) normal (0, 1, 0) x (-1, 0, 0)
  line L0 (11.7, 10) -> (16.5, 10)
  line L1 (16.5, 10) -> (16.5, 23)
  line L2 (16.5, 23) -> (11.7, 23)
  line L3 (11.7, 23) -> (11.7, 10)
  line L4 (14.1, 10) -> (14.1, 16.25) construction
  circle A0 centre (14.1, 16.25) radius 1.4
  dimension "d107" = 6.25
  dimension "d108" = 2.8
  constraint midpoint L0 L4.start
  constraint perpendicular L0 L4
  constraint coincident L4.end A0.centre
  measures "d107" distance of L4.start L4.end
  measures "d108" diameter of A0
extrude "Extrude16" cut sketch "Sketch16" sketch "Sketch15" against normal blind 4.475 contours A0 of sketch 2 contours A0
sketch "Sketch17" plane through (0, -16.5, 0) normal (0, -1, 0) x (1, 0, 0)
  line L0 (-16.5, 10) -> (16.5, 10)
  line L1 (16.5, 10) -> (16.5, 23)
  line L2 (16.5, 23) -> (-16.5, 23)
  line L3 (-16.5, 23) -> (-16.5, 10)
  line L4 (-16.5, 10) -> (16.5, 23) construction
  line L5 (16.5, 10) -> (-16.5, 23) construction
  line L6 (0, 16.5) -> (-5.7, 16.5) construction
  circle A0 centre (-5.7, 16.5) radius 2.5
  dimension "d120" = 5.7
  dimension "d121" = 5
  constraint coincident L0.start L3.end
  constraint coincident L1.end L2.start
  constraint coincident L0.end L1.start
  constraint coincident L2.end L3.start
  constraint horizontal L6
  constraint coincident L6.end A0.centre
  measures "d120" distance of L6.start L6.end
  measures "d121" diameter of A0
extrude "Extrude17" add sketch "Sketch17" along normal blind 3.5 contours A0
fillet "Fillet8" radius 2.5 1 faces at (-6.4508, -20, 16.1384)
fillet "Fillet9" radius 1 4 edges at (16.5, -16.5, 16.5) (-16.5, -16.5, 16.5) (-16.5, 11.5, 16.5) (16.5, 11.5, 16.5)
fillet "Fillet10" radius 2.5 2 edges at (-23.3082, -9.0404, 10) (-23.3082, -9.0404, 0)
equation "fullServoLength = 32.45 mm"
